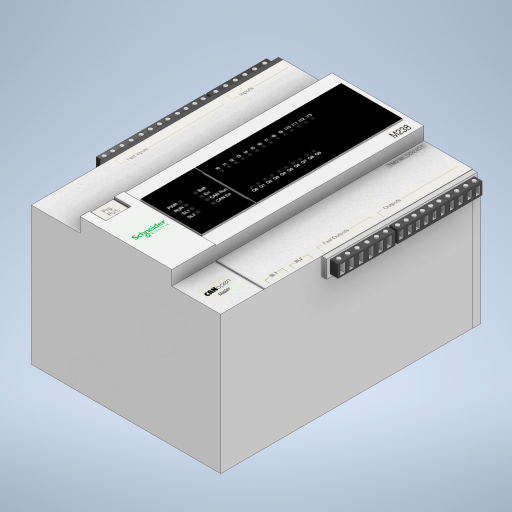
# Autodesk Inventor part: PLC
Saved by Autodesk Inventor 2023 (Build 270158000, 158)
## iProperties
Created: 2022-07-08
Part Number: PLC
Material: Generic
Document SubType Name: Sheet Metal
Designer: User
Density: 1 g/cm^3
Sheet Metal Rule: Default
Appearance: Default
Author: User
Autodesk Inventor part; units mm, degrees
ref_plane "YZ Plane" through (0, 0, 0) normal (1, 0, 0) x (0, 1, 0)
ref_plane "XZ Plane" through (0, 0, 0) normal (0, 1, 0) x (-1, 0, 0)
ref_plane "XY Plane" through (0, 0, 0) normal (0, 0, 1) x (1, 0, 0)
sketch "Sketch1" plane through (0, 0, 0) normal (0, 1, 0) x (-1, 0, 0)
  line L0 (-59, -78.5) -> (59, -78.5)
  line L1 (59, -78.5) -> (59, 78.5)
  line L2 (59, 78.5) -> (-59, 78.5)
  line L3 (-59, 78.5) -> (-59, -78.5)
  line L4 (-59, -78.5) -> (59, 78.5) construction
  line L5 (59, -78.5) -> (-59, 78.5) construction
  point P0 (0, 0)
  constraints: 12 end point, 2 midpoint, 2 parallel, 1 horizontal, 1 perpendicular
extrude "Extrusion1" add sketch "Sketch1" along normal blind 86
sketch "Sketch2" plane through (0, 86, 0) normal (0, 1, 0) x (1, 0, 0)
  line L0 (-59, -78.5) -> (59, -78.5) projected
  line L1 (28.5872, 78.5) -> (-28.5872, 78.5)
  line L2 (-28.5872, 78.5) -> (-28.5872, -78.5)
  line L3 (-28.5872, -78.5) -> (28.5872, -78.5)
  line L4 (28.5872, -78.5) -> (28.5872, 78.5)
  line L5 (28.5872, 78.5) -> (-28.5872, -78.5) construction
  line L6 (-28.5872, 78.5) -> (28.5872, -78.5) construction
  point P0 (0, 0)
  constraints: 12 end point, 2 midpoint, 2 parallel, 1 horizontal, 1 perpendicular, 1 point on line
extrude "Extrusion2" add sketch "Sketch2" along normal blind 8
sketch "Sketch3" plane through (0, 94, 0) normal (0, 1, 0) x (1, 0, 0)
  line L0 (-28.5872, 78.5) -> (-28.5872, -78.5) projected
  line L1 (28.5872, -51.4185) -> (-28.5872, -51.4185)
  line L2 (-28.5872, -51.4185) -> (-28.5872, -78.5)
  line L3 (-28.5872, -78.5) -> (28.5872, -78.5)
  line L4 (28.5872, -78.5) -> (28.5872, -51.4185)
  line L5 (28.5872, -51.4185) -> (-28.5872, -78.5) construction
  line L6 (-28.5872, -51.4185) -> (28.5872, -78.5) construction
  line L7 (-19.1432, -51.4185) -> (19.1432, -51.4185)
  line L8 (18.8938, 74.8007) -> (-19.149, 74.8007)
  line L9 (-19.149, 74.8007) -> (-19.149, -16.0949)
  line L10 (-19.149, -16.0949) -> (18.8938, -16.0949)
  line L11 (18.8938, -16.0949) -> (18.8938, 74.8007)
  line L12 (18.8938, 74.8007) -> (-19.149, -16.0949) construction
  line L13 (-19.149, 74.8007) -> (18.8938, -16.0949) construction
  line L14 (18.8938, -16.7205) -> (-19.149, -16.7205)
  line L15 (-19.149, -16.7205) -> (-19.149, -50.1614)
  line L16 (-19.149, -50.1614) -> (18.8938, -50.1614)
  line L17 (18.8938, -50.1614) -> (18.8938, -16.7205)
  line L18 (18.8938, -16.7205) -> (-19.149, -50.1614) construction
  line L19 (-19.149, -16.7205) -> (18.8938, -50.1614) construction
  point P0 (0, 0)
  point P1 (0, -64.9593)
  point P2 (-0.1276, 29.3529)
  point P3 (-0.1276, -33.4409)
  constraints: 38 end point, 6 midpoint, 6 parallel, 3 horizontal, 3 perpendicular, 1 point on line
extrude "Extrusion3" add sketch "Sketch3" along normal blind 1 contours L11 L10 L9 L8
extrude "Extrusion4" add sketch "Sketch3" along normal blind 1 contours L17 L16 L15 L14
extrude "Extrusion5" add sketch "Sketch3" along normal blind 1 contours L1 L4 L3 L0
sketch "Sketch4" plane through (0, 95, 0) normal (0, 1, 0) x (1, 0, 0)
  line L0 (-28.5872, -78.5) -> (-28.5872, 78.5) projected
  line L1 (-18.1707, -57.2784) -> (-28.5872, -57.2784)
  line L2 (-28.5872, -57.2784) -> (-28.5872, -72.8644)
  line L3 (-28.5872, -72.8644) -> (-18.1707, -72.8644)
  line L4 (-18.1707, -72.8644) -> (-18.1707, -57.2784)
  line L5 (-18.1707, -57.2784) -> (-28.5872, -72.8644) construction
  line L6 (-28.5872, -57.2784) -> (-18.1707, -72.8644) construction
  point P0 (0, 0)
  point P1 (-23.379, -65.0714)
  constraints: 12 end point, 2 midpoint, 2 parallel, 1 horizontal, 1 perpendicular, 1 point on line
extrude "Extrusion6" cut sketch "Sketch4" against normal blind 1
sketch "Sketch5" plane through (-59, 0, -78.5) normal (-1, 0, 0) x (0, 0, 1)
  line L0 (-0.0793, 85.7228) -> (111.1007, 85.7228)
  line L1 (111.1007, 85.7228) -> (111.1007, 74.8127)
  line L2 (111.1007, 74.8127) -> (-0.0793, 74.8127)
  line L3 (-0.0793, 74.8127) -> (-0.0793, 85.7228)
  line L4 (-0.0793, 85.7228) -> (111.1007, 74.8127) construction
  line L5 (111.1007, 85.7228) -> (-0.0793, 74.8127) construction
  point P0 (78.5, 0)
  point P1 (55.5107, 80.2677)
  dimension "d270" = 10.9102
  constraints: 12 end point, 2 midpoint, 2 parallel, 1 horizontal, 1 perpendicular
  measures "d270" distance of L0.end L1.end
extrude "Extrusion7" add sketch "Sketch5" along normal blind 3
sketch "Sketch6" plane through (-62, 0, -78.5) normal (-1, 0, 0) x (0, 0, 1)
  line L0 (40.9569, 76.775) -> (108.5085, 76.775)
  line L1 (108.5085, 76.775) -> (108.5085, 83.79)
  line L2 (108.5085, 83.79) -> (40.9569, 83.79)
  line L3 (40.9569, 83.79) -> (40.9569, 76.775)
  line L4 (40.9569, 76.775) -> (108.5085, 83.79) construction
  line L5 (108.5085, 76.775) -> (40.9569, 83.79) construction
  line L6 (2.4823, 83.7437) -> (39.9398, 83.7437)
  line L7 (39.9398, 83.7437) -> (39.9398, 76.8213)
  line L8 (39.9398, 76.8213) -> (2.4823, 76.8213)
  line L9 (2.4823, 76.8213) -> (2.4823, 83.7437)
  line L10 (2.4823, 83.7437) -> (39.9398, 76.8213) construction
  line L11 (39.9398, 83.7437) -> (2.4823, 76.8213) construction
  point P0 (78.5, 0)
  point P1 (74.7327, 80.2825)
  point P2 (21.211, 80.2825)
  constraints: 24 end point, 4 midpoint, 4 parallel, 2 horizontal, 2 perpendicular
extrude "Extrusion8" add sketch "Sketch6" along normal blind 5 contours L3 L2 L1 L0
extrude "Extrusion9" add sketch "Sketch6" along normal blind 5 contours L6 L7 L8 L9
sketch "Sketch7" plane through (-62, 83.79, 30.0085) normal (0, 1, 0) x (1, 0, 0)
  circle A0 centre (-2.5704, 2.5116) radius 1.27
  circle A1 centre (-2.5676, 7.7493) radius 1.27
  circle A2 centre (-2.5676, 19.2576) radius 1.27
  circle A3 centre (-2.5676, 13.5035) radius 1.27
  circle A4 centre (-2.5676, 25.5282) radius 1.27
  circle A5 centre (-2.5676, 31.3561) radius 1.27
  circle A6 centre (-2.5676, 42.1267) radius 1.27
  circle A7 centre (-2.5676, 36.9627) radius 1.27
  circle A8 centre (-2.5676, 48.1759) radius 1.27
  circle A9 centre (-2.5676, 53.4874) radius 1.27
  circle A10 centre (-2.5676, 64.1678) radius 1.27
  circle A11 centre (-2.5676, 58.9465) radius 1.27
  point P0 (62, 30.0085)
  dimension "d20" = 2.54
  dimension "d21" = 2.54
  dimension "d22" = 2.54
  dimension "d23" = 2.54
  dimension "d24" = 2.54
  dimension "d25" = 2.54
  dimension "d26" = 2.54
  dimension "d27" = 2.54
  dimension "d28" = 2.54
  dimension "d29" = 2.54
  dimension "d30" = 2.54
  dimension "d31" = 2.54
  constraints: 12 centre point
  measures "d20" diameter of A0
  measures "d21" diameter of A1
  measures "d22" diameter of A2
  measures "d23" diameter of A3
  measures "d24" diameter of A4
  measures "d25" diameter of A5
  measures "d26" diameter of A6
  measures "d27" diameter of A7
  measures "d28" diameter of A8
  measures "d29" diameter of A9
  measures "d30" diameter of A10
  measures "d31" diameter of A11
extrude "Extrusion10" add sketch "Sketch7" along normal blind 0.5 contours A0
extrude "Extrusion11" add sketch "Sketch7" along normal blind 0.5 contours A1
extrude "Extrusion12" add sketch "Sketch7" along normal blind 0.5 contours A3
extrude "Extrusion13" add sketch "Sketch7" along normal blind 0.5 contours A2
extrude "Extrusion14" add sketch "Sketch7" along normal blind 0.5 contours A4
extrude "Extrusion15" add sketch "Sketch7" along normal blind 0.5 contours A5
extrude "Extrusion16" add sketch "Sketch7" along normal blind 0.5 contours A7
extrude "Extrusion17" add sketch "Sketch7" along normal blind 0.5 contours A6
extrude "Extrusion18" add sketch "Sketch7" along normal blind 0.5 contours A8
extrude "Extrusion19" add sketch "Sketch7" along normal blind 0.5 contours A9
extrude "Extrusion20" add sketch "Sketch7" along normal blind 0.5 contours A11
extrude "Extrusion21" add sketch "Sketch7" along normal blind 0.5 contours A10
sketch "Sketch8" plane through (-62, 83.7437, -38.5602) normal (0, 1, 0) x (1, 0, 0)
  circle A0 centre (-2.5305, 3.4573) radius 1.27
  circle A1 centre (-2.5952, 9.6724) radius 1.27
  circle A2 centre (-2.5952, 21.6396) radius 1.27
  circle A3 centre (-2.5952, 15.689) radius 1.27
  circle A4 centre (-2.5952, 27.7224) radius 1.27
  circle A5 centre (-2.5952, 34.0035) radius 1.27
  point P0 (62, -38.5602)
  dimension "d56" = 2.54
  dimension "d57" = 2.54
  dimension "d58" = 2.54
  dimension "d59" = 2.54
  dimension "d60" = 2.54
  dimension "d61" = 2.54
  constraints: 6 centre point
  measures "d56" diameter of A0
  measures "d57" diameter of A1
  measures "d58" diameter of A2
  measures "d59" diameter of A3
  measures "d60" diameter of A4
  measures "d61" diameter of A5
extrude "Extrusion22" add sketch "Sketch8" along normal blind 0.5 contours A0
extrude "Extrusion23" add sketch "Sketch8" along normal blind 0.5 contours A1
extrude "Extrusion24" add sketch "Sketch8" along normal blind 0.5 contours A3
extrude "Extrusion25" add sketch "Sketch8" along normal blind 0.5 contours A2
extrude "Extrusion26" add sketch "Sketch8" along normal blind 0.5 contours A4
extrude "Extrusion27" add sketch "Sketch8" along normal blind 0.5 contours A5
sketch "Sketch9" plane through (0, 95, 0) normal (0, 1, 0) x (1, 0, 0)
  line L0 (-10.1047, -53.1992) -> (11.9504, -53.1992) construction
  line L1 (11.9504, -53.1992) -> (11.9504, -75.483) construction
  line L2 (11.9504, -75.483) -> (-10.1047, -75.483) construction
  line L3 (-10.1047, -75.483) -> (-10.1047, -53.1992) construction
  point P0 (0, 0)
  constraints: 2 other
decal "Decal1"
sketch "Sketch10" plane through (0, 95, 0) normal (0, 1, 0) x (1, 0, 0)
  line L0 (-13.6554, -16.7848) -> (14.4275, -16.7848) construction
  line L1 (14.4275, -16.7848) -> (14.4275, -50.0682) construction
  line L2 (14.4275, -50.0682) -> (-13.6554, -50.0682) construction
  line L3 (-13.6554, -50.0682) -> (-13.6554, -16.7848) construction
  line L4 (21.6211, 74.4866) -> (26.8689, 74.4866) construction
  line L5 (26.8689, 74.4866) -> (26.8689, 61.9983) construction
  line L6 (26.8689, 61.9983) -> (21.6211, 61.9983) construction
  line L7 (21.6211, 61.9983) -> (21.6211, 74.4866) construction
  line L8 (-58.2252, 36.6989) -> (-51.617, 36.6989) construction
  line L9 (-51.617, 36.6989) -> (-51.617, -29.4508) construction
  line L10 (-51.617, -29.4508) -> (-58.2252, -29.4508) construction
  line L11 (-58.2252, -29.4508) -> (-58.2252, 36.6989) construction
  point P0 (0, 0)
  constraints: 6 other
decal "Decal2"
decal "Decal3"
decal "Decal4"
sketch "Sketch11" plane through (0, 86, 0) normal (0, 1, 0) x (1, 0, 0)
  line L0 (29.6735, 76.7479) -> (33.1381, 76.7479) construction
  line L1 (33.1381, 76.7479) -> (33.1381, 52.8308) construction
  line L2 (33.1381, 52.8308) -> (29.6735, 52.8308) construction
  line L3 (29.6735, 52.8308) -> (29.6735, 76.7479) construction
  point P0 (0, 0)
  constraints: 2 other
decal "Decal5"
sketch "Sketch12" plane through (0, 86, 0) normal (0, 1, 0) x (1, 0, 0)
  line L0 (-58.554, 77.2781) -> (-50.311, 77.2781) construction
  line L1 (-50.311, 77.2781) -> (-50.311, 39.3956) construction
  line L2 (-50.311, 39.3956) -> (-58.554, 39.3956) construction
  line L3 (-58.554, 39.3956) -> (-58.554, 77.2781) construction
  point P0 (0, 0)
  constraints: 2 other
decal "Decal6"
sketch "Sketch13" plane through (59, 0, 78.5) normal (1, 0, 0) x (0, 0, -1)
  line L0 (156.8045, 74.8146) -> (63.0543, 74.8146)
  line L1 (63.0543, 74.8146) -> (63.0543, 85.7366)
  line L2 (63.0543, 85.7366) -> (156.8045, 85.7366)
  line L3 (156.8045, 85.7366) -> (156.8045, 74.8146)
  line L4 (156.8045, 74.8146) -> (63.0543, 85.7366) construction
  line L5 (63.0543, 74.8146) -> (156.8045, 85.7366) construction
  point P0 (78.5, 0)
  point P1 (109.9294, 80.2756)
  constraints: 12 end point, 2 midpoint, 2 parallel, 1 horizontal, 1 perpendicular
extrude "Extrusion28" add sketch "Sketch13" along normal blind 3
sketch "Sketch14" plane through (62, 86, 0) normal (1, 0, 0) x (0, -1, 0)
  line L0 (9.3005, -13.3278) -> (1.4582, -13.3278)
  line L1 (1.4582, -13.3278) -> (1.4582, 22.2214)
  line L2 (1.4582, 22.2214) -> (9.3005, 22.2214)
  line L3 (9.3005, 22.2214) -> (9.3005, -13.3278)
  line L4 (9.3005, -13.3278) -> (1.4582, 22.2214) construction
  line L5 (1.4582, -13.3278) -> (9.3005, 22.2214) construction
  line L6 (1.5726, 23.7364) -> (9.1861, 23.7364)
  line L7 (9.1861, 23.7364) -> (9.1861, 76.506)
  line L8 (9.1861, 76.506) -> (1.5726, 76.506)
  line L9 (1.5726, 76.506) -> (1.5726, 23.7364)
  line L10 (1.5726, 23.7364) -> (9.1861, 76.506) construction
  line L11 (9.1861, 23.7364) -> (1.5726, 76.506) construction
  point P0 (86, 0)
  point P1 (5.3794, 4.4468)
  point P2 (5.3794, 50.1212)
  constraints: 24 end point, 4 midpoint, 4 parallel, 2 horizontal, 2 perpendicular
extrude "Extrusion29" add sketch "Sketch14" along normal blind 5 contours L0 L1 L2 L3
extrude "Extrusion30" add sketch "Sketch14" along normal blind 5 contours L9 L8 L7 L6
sketch "Sketch15" plane through (62, 84.5418, 13.3278) normal (0, 1, 0) x (1, 0, 0)
  circle A0 centre (2.4904, 2.9128) radius 1.27
  circle A1 centre (2.4904, 8.3521) radius 1.27
  circle A2 centre (2.4904, 14.2858) radius 1.27
  circle A3 centre (2.4904, 20.4668) radius 1.27
  circle A4 centre (2.4904, 26.4006) radius 1.27
  circle A5 centre (2.4904, 32.0253) radius 1.27
  point P0 (-62, 13.3278)
  dimension "d278" = 2.54
  dimension "d279" = 2.54
  dimension "d280" = 2.54
  dimension "d281" = 2.54
  dimension "d282" = 2.54
  dimension "d283" = 2.54
  constraints: 6 centre point
  measures "d278" diameter of A0
  measures "d279" diameter of A1
  measures "d280" diameter of A2
  measures "d281" diameter of A3
  measures "d282" diameter of A4
  measures "d283" diameter of A5
extrude "Extrusion31" add sketch "Sketch15" along normal blind 0.5 contours A0
extrude "Extrusion32" add sketch "Sketch15" along normal blind 0.5 contours A1
extrude "Extrusion33" add sketch "Sketch15" along normal blind 0.5 contours A2
extrude "Extrusion34" add sketch "Sketch15" along normal blind 0.5 contours A3
extrude "Extrusion35" add sketch "Sketch15" along normal blind 0.5 contours A4
extrude "Extrusion36" add sketch "Sketch15" along normal blind 0.5 contours A5
sketch "Sketch16" plane through (62, 84.4274, -23.7364) normal (0, 1, 0) x (1, 0, 0)
  circle A0 centre (2.6563, 2.3164) radius 1.27
  circle A1 centre (2.6563, 7.6321) radius 1.27
  circle A2 centre (2.6563, 12.5769) radius 1.27
  circle A3 centre (2.6563, 17.7689) radius 1.27
  circle A4 centre (2.6563, 22.8991) radius 1.27
  circle A5 centre (2.6563, 28.0912) radius 1.27
  circle A6 centre (2.6563, 33.5922) radius 1.27
  circle A7 centre (2.6563, 39.1551) radius 1.27
  circle A8 centre (2.6563, 44.7798) radius 1.27
  circle A9 centre (2.6563, 50.0337) radius 1.27
  point P0 (-62, -23.7364)
  dimension "d296" = 2.54
  dimension "d297" = 2.54
  dimension "d298" = 2.54
  dimension "d299" = 2.54
  dimension "d300" = 2.54
  dimension "d301" = 2.54
  dimension "d302" = 2.54
  dimension "d303" = 2.54
  dimension "d304" = 2.54
  dimension "d305" = 2.54
  constraints: 10 centre point
  measures "d296" diameter of A0
  measures "d297" diameter of A1
  measures "d298" diameter of A2
  measures "d299" diameter of A3
  measures "d300" diameter of A4
  measures "d301" diameter of A5
  measures "d302" diameter of A6
  measures "d303" diameter of A7
  measures "d304" diameter of A8
  measures "d305" diameter of A9
extrude "Extrusion37" add sketch "Sketch16" along normal blind 0.5 contours A0
extrude "Extrusion38" add sketch "Sketch16" along normal blind 0.5 contours A1
extrude "Extrusion39" add sketch "Sketch16" along normal blind 0.5 contours A2
extrude "Extrusion40" add sketch "Sketch16" along normal blind 0.5 contours A3
extrude "Extrusion41" add sketch "Sketch16" along normal blind 0.5 contours A4
extrude "Extrusion42" add sketch "Sketch16" along normal blind 0.5 contours A5
extrude "Extrusion43" add sketch "Sketch16" along normal blind 0.5 contours A6
extrude "Extrusion44" add sketch "Sketch16" along normal blind 0.5 contours A7
extrude "Extrusion45" add sketch "Sketch16" along normal blind 0.5 contours A8
extrude "Extrusion46" add sketch "Sketch16" along normal blind 0.5 contours A9
sketch "Sketch17" plane through (0, 86, 0) normal (0, 1, 0) x (1, 0, 0)
  line L0 (50.4208, 77.1669) -> (57.9021, 77.1669) construction
  line L1 (57.9021, 77.1669) -> (57.9021, 23.3015) construction
  line L2 (57.9021, 23.3015) -> (50.4208, 23.3015) construction
  line L3 (50.4208, 23.3015) -> (50.4208, 77.1669) construction
  line L4 (50.1649, 22.395) -> (58.1661, 22.395) construction
  line L5 (58.1661, 22.395) -> (58.1661, -14.0662) construction
  line L6 (58.1661, -14.0662) -> (50.1649, -14.0662) construction
  line L7 (50.1649, -14.0662) -> (50.1649, 22.395) construction
  point P0 (0, 0)
  constraints: 4 other
decal "Decal7"
decal "Decal8"
sketch "Sketch18" plane through (0, 95, 0) normal (0, 1, 0) x (1, 0, 0)
  line L0 (-16.2341, 72.1064) -> (15.9464, 72.1064) construction
  line L1 (15.9464, 72.1064) -> (15.9464, -14.584) construction
  line L2 (15.9464, -14.584) -> (-16.2341, -14.584) construction
  line L3 (-16.2341, -14.584) -> (-16.2341, 72.1064) construction
  point P0 (0, 0)
  constraints: 2 other
decal "Decal9"
sketch "Sketch19" plane through (59, 0, -78.5) normal (0, 0, -1) x (-1, 0, 0)
  line L0 (0.0162, 74.5415) -> (117.9838, 74.5415)
  line L1 (117.9838, 74.5415) -> (117.9838, -0.0836)
  line L2 (117.9838, -0.0836) -> (0.0162, -0.0836)
  line L3 (0.0162, -0.0836) -> (0.0162, 74.5415)
  line L4 (0.0162, 74.5415) -> (117.9838, -0.0836) construction
  line L5 (117.9838, 74.5415) -> (0.0162, -0.0836) construction
  point P0 (59, 0)
  point P1 (59, 37.229)
  constraints: 12 end point, 2 midpoint, 2 parallel, 1 horizontal, 1 perpendicular
extrude "Extrusion47" add sketch "Sketch19" along normal blind 5
sketch "Sketch20" plane through (-67, 0, -78.5) normal (-1, 0, 0) x (0, 0, 1)
  line L0 (107.1255, 82.555) -> (104.7702, 82.555)
  line L1 (104.7702, 82.555) -> (104.7702, 78.0406)
  line L2 (104.7702, 78.0406) -> (107.1255, 78.0406)
  line L3 (107.1255, 78.0406) -> (107.1255, 82.555)
  line L4 (107.1255, 82.555) -> (104.7702, 78.0406) construction
  line L5 (104.7702, 82.555) -> (107.1255, 78.0406) construction
  line L6 (102.2296, 78.0852) -> (99.7509, 78.0852)
  line L7 (99.7509, 78.0852) -> (99.7509, 82.5104)
  line L8 (99.7509, 82.5104) -> (102.2296, 82.5104)
  line L9 (102.2296, 82.5104) -> (102.2296, 78.0852)
  line L10 (102.2296, 78.0852) -> (99.7509, 82.5104) construction
  line L11 (99.7509, 78.0852) -> (102.2296, 82.5104) construction
  line L12 (96.3367, 78.063) -> (93.6848, 78.063)
  line L13 (93.6848, 78.063) -> (93.6848, 82.5326)
  line L14 (93.6848, 82.5326) -> (96.3367, 82.5326)
  line L15 (96.3367, 82.5326) -> (96.3367, 78.063)
  line L16 (96.3367, 78.063) -> (93.6848, 82.5326) construction
  line L17 (93.6848, 78.063) -> (96.3367, 82.5326) construction
  line L18 (90.8512, 78.0898) -> (88.1425, 78.0898)
  line L19 (88.1425, 78.0898) -> (88.1425, 82.5058)
  line L20 (88.1425, 82.5058) -> (90.8512, 82.5058)
  line L21 (90.8512, 82.5058) -> (90.8512, 78.0898)
  line L22 (90.8512, 78.0898) -> (88.1425, 82.5058) construction
  line L23 (88.1425, 78.0898) -> (90.8512, 82.5058) construction
  line L24 (84.4554, 78.0406) -> (81.7075, 78.0406)
  line L25 (81.7075, 78.0406) -> (81.7075, 82.555)
  line L26 (81.7075, 82.555) -> (84.4554, 82.555)
  line L27 (84.4554, 82.555) -> (84.4554, 78.0406)
  line L28 (84.4554, 78.0406) -> (81.7075, 82.555) construction
  line L29 (81.7075, 78.0406) -> (84.4554, 82.555) construction
  line L30 (78.5647, 82.744) -> (75.8543, 82.744)
  line L31 (75.8543, 82.744) -> (75.8543, 78.3053)
  line L32 (75.8543, 78.3053) -> (78.5647, 78.3053)
  line L33 (78.5647, 78.3053) -> (78.5647, 82.744)
  line L34 (78.5647, 82.744) -> (75.8543, 78.3053) construction
  line L35 (75.8543, 82.744) -> (78.5647, 78.3053) construction
  line L36 (73.1672, 78.1595) -> (70.2252, 78.1595)
  line L37 (70.2252, 78.1595) -> (70.2252, 82.744)
  line L38 (70.2252, 82.744) -> (73.1672, 82.744)
  line L39 (73.1672, 82.744) -> (73.1672, 78.1595)
  line L40 (73.1672, 78.1595) -> (70.2252, 82.744) construction
  line L41 (70.2252, 78.1595) -> (73.1672, 82.744) construction
  line L42 (65.4366, 82.5982) -> (67.8698, 82.5982)
  line L43 (67.8698, 82.5982) -> (67.8698, 78.3053)
  line L44 (67.8698, 78.3053) -> (65.4366, 78.3053)
  line L45 (65.4366, 78.3053) -> (65.4366, 82.5982)
  line L46 (65.4366, 82.5982) -> (67.8698, 78.3053) construction
  line L47 (67.8698, 82.5982) -> (65.4366, 78.3053) construction
  line L48 (59.1355, 82.5982) -> (61.6871, 82.5982)
  line L49 (61.6871, 82.5982) -> (61.6871, 78.3053)
  line L50 (61.6871, 78.3053) -> (59.1355, 78.3053)
  line L51 (59.1355, 78.3053) -> (59.1355, 82.5982)
  line L52 (59.1355, 82.5982) -> (61.6871, 78.3053) construction
  line L53 (61.6871, 82.5982) -> (59.1355, 78.3053) construction
  line L54 (48.5435, 82.8095) -> (51.0951, 82.8095)
  line L55 (51.0951, 82.8095) -> (51.0951, 78.4731)
  line L56 (51.0951, 78.4731) -> (48.5435, 78.4731)
  line L57 (48.5435, 78.4731) -> (48.5435, 82.8095)
  line L58 (48.5435, 82.8095) -> (51.0951, 78.4731) construction
  line L59 (51.0951, 82.8095) -> (48.5435, 78.4731) construction
  line L60 (43.0921, 82.7647) -> (45.5408, 82.7647)
  line L61 (45.5408, 82.7647) -> (45.5408, 78.5179)
  line L62 (45.5408, 78.5179) -> (43.0921, 78.5179)
  line L63 (43.0921, 78.5179) -> (43.0921, 82.7647)
  line L64 (43.0921, 82.7647) -> (45.5408, 78.5179) construction
  line L65 (45.5408, 82.7647) -> (43.0921, 78.5179) construction
  line L66 (56.2786, 76.6995) -> (56.2786, 84.5418) projected
  line L67 (53.2485, 82.7234) -> (56.2786, 82.7234)
  line L68 (56.2786, 82.7234) -> (56.2786, 78.5179)
  line L69 (56.2786, 78.5179) -> (53.2485, 78.5179)
  line L70 (53.2485, 78.5179) -> (53.2485, 82.7234)
  line L71 (54.7636, 84.4274) -> (54.7636, 76.8139) projected
  line L72 (53.2485, 82.7234) -> (56.2786, 78.5179) construction
  line L73 (56.2786, 82.7234) -> (53.2485, 78.5179) construction
  point P0 (78.5, 0)
  point P1 (105.9478, 80.2978)
  point P2 (100.9903, 80.2978)
  point P3 (95.0108, 80.2978)
  point P4 (89.4968, 80.2978)
  point P5 (83.0814, 80.2978)
  point P6 (77.2095, 80.5246)
  point P7 (71.6962, 80.4517)
  point P8 (66.6532, 80.4517)
  point P9 (60.4113, 80.4517)
  point P10 (49.8193, 80.6413)
  point P11 (44.3165, 80.6413)
  point P12 (54.7636, 80.6206)
  point P13 (54.7636, 78.5179)
  point P14 (54.7636, 82.7234)
  constraints: 144 end point, 25 midpoint, 24 parallel, 12 horizontal, 12 perpendicular, 2 point on line
extrude "Extrusion48" cut sketch "Sketch20" against normal blind 4 contours L3 L2 L1 L0
extrude "Extrusion49" cut sketch "Sketch20" against normal blind 4 contours L6 L7 L8 L9
extrude "Extrusion50" cut sketch "Sketch20" against normal blind 4 contours L12 L13 L14 L15
extrude "Extrusion51" cut sketch "Sketch20" against normal blind 4 contours L18 L19 L20 L21
extrude "Extrusion52" cut sketch "Sketch20" against normal blind 4 contours L24 L25 L26 L27
extrude "Extrusion53" cut sketch "Sketch20" against normal blind 4 contours L33 L32 L31 L30
extrude "Extrusion54" cut sketch "Sketch20" against normal blind 4 contours L36 L37 L38 L39
extrude "Extrusion55" cut sketch "Sketch20" against normal blind 4 contours L42 L43 L44 L45
extrude "Extrusion56" cut sketch "Sketch20" against normal blind 4 contours L48 L49 L50 L51
extrude "Extrusion57" cut sketch "Sketch20" against normal blind 4 contours L69 L70 L67 L71
extrude "Extrusion58" cut sketch "Sketch20" against normal blind 4 contours L69 L71 L67 L66
extrude "Extrusion59" cut sketch "Sketch20" against normal blind 4 contours L54 L55 L56 L57
extrude "Extrusion60" cut sketch "Sketch20" against normal blind 4 contours L60 L61 L62 L63
sketch "Sketch21" plane through (-67, 0, -78.5) normal (-1, 0, 0) x (0, 0, 1)
  line L0 (35.0939, 83.0672) -> (37.8762, 83.0672)
  line L1 (37.8762, 83.0672) -> (37.8762, 77.7742)
  line L2 (37.8762, 77.7742) -> (35.0939, 77.7742)
  line L3 (35.0939, 77.7742) -> (35.0939, 83.0672)
  line L4 (35.0939, 83.0672) -> (37.8762, 77.7742) construction
  line L5 (37.8762, 83.0672) -> (35.0939, 77.7742) construction
  line L6 (31.7697, 77.7742) -> (28.9875, 77.7742)
  line L7 (28.9875, 77.7742) -> (28.9875, 83.0672)
  line L8 (28.9875, 83.0672) -> (31.7697, 83.0672)
  line L9 (31.7697, 83.0672) -> (31.7697, 77.7742)
  line L10 (31.7697, 77.7742) -> (28.9875, 83.0672) construction
  line L11 (28.9875, 77.7742) -> (31.7697, 83.0672) construction
  line L12 (25.5597, 77.7742) -> (23.0489, 77.7742)
  line L13 (23.0489, 77.7742) -> (23.0489, 83.0672)
  line L14 (23.0489, 83.0672) -> (25.5597, 83.0672)
  line L15 (25.5597, 83.0672) -> (25.5597, 77.7742)
  line L16 (25.5597, 77.7742) -> (23.0489, 83.0672) construction
  line L17 (23.0489, 77.7742) -> (25.5597, 83.0672) construction
  line L18 (19.622, 77.7742) -> (16.9755, 77.7742)
  line L19 (16.9755, 77.7742) -> (16.9755, 83.0672)
  line L20 (16.9755, 83.0672) -> (19.622, 83.0672)
  line L21 (19.622, 83.0672) -> (19.622, 77.7742)
  line L22 (19.622, 77.7742) -> (16.9755, 83.0672) construction
  line L23 (16.9755, 77.7742) -> (19.622, 83.0672) construction
  line L24 (13.6504, 77.7742) -> (11.0039, 77.7742)
  line L25 (11.0039, 77.7742) -> (11.0039, 83.0672)
  line L26 (11.0039, 83.0672) -> (13.6504, 83.0672)
  line L27 (13.6504, 83.0672) -> (13.6504, 77.7742)
  line L28 (13.6504, 77.7742) -> (11.0039, 83.0672) construction
  line L29 (11.0039, 77.7742) -> (13.6504, 83.0672) construction
  line L30 (7.3395, 77.7742) -> (4.6251, 77.7742)
  line L31 (4.6251, 77.7742) -> (4.6251, 83.0672)
  line L32 (4.6251, 83.0672) -> (7.3395, 83.0672)
  line L33 (7.3395, 83.0672) -> (7.3395, 77.7742)
  line L34 (7.3395, 77.7742) -> (4.6251, 83.0672) construction
  line L35 (4.6251, 77.7742) -> (7.3395, 83.0672) construction
  point P0 (78.5, 0)
  point P1 (36.485, 80.4207)
  point P2 (30.3786, 80.4207)
  point P3 (24.3043, 80.4207)
  point P4 (18.2988, 80.4207)
  point P5 (12.3272, 80.4207)
  point P6 (5.9823, 80.4207)
  constraints: 72 end point, 12 midpoint, 12 parallel, 6 horizontal, 6 perpendicular, 3 point on line
extrude "Extrusion61" cut sketch "Sketch21" against normal blind 4 contours L0 L1 L2 L3
extrude "Extrusion62" cut sketch "Sketch21" against normal blind 4 contours L6 L7 L8 L9
extrude "Extrusion63" cut sketch "Sketch21" against normal blind 4 contours L12 L13 L14 L15
extrude "Extrusion64" cut sketch "Sketch21" against normal blind 4 contours L18 L19 L20 L21
extrude "Extrusion65" cut sketch "Sketch21" against normal blind 4 contours L24 L25 L26 L27
extrude "Extrusion66" cut sketch "Sketch21" against normal blind 4 contours L30 L31 L32 L33
sketch "Sketch22" plane through (67, 86, 0) normal (1, 0, 0) x (0, 0, -1)
  line L0 (-11.9749, -2.376) -> (-8.9475, -2.376)
  line L1 (-8.9475, -2.376) -> (-8.9475, -8.4309)
  line L2 (-8.9475, -8.4309) -> (-11.9749, -8.4309)
  line L3 (-11.9749, -8.4309) -> (-11.9749, -2.376)
  line L4 (-11.9749, -2.376) -> (-8.9475, -8.4309) construction
  line L5 (-8.9475, -2.376) -> (-11.9749, -8.4309) construction
  line L6 (-6.5226, -2.376) -> (-3.5286, -2.376)
  line L7 (-3.5286, -2.376) -> (-3.5286, -8.4309)
  line L8 (-3.5286, -8.4309) -> (-6.5226, -8.4309)
  line L9 (-6.5226, -8.4309) -> (-6.5226, -2.376)
  line L10 (-6.5226, -2.376) -> (-3.5286, -8.4309) construction
  line L11 (-3.5286, -2.376) -> (-6.5226, -8.4309) construction
  line L12 (-0.3577, -2.3822) -> (2.5081, -2.3822)
  line L13 (2.5081, -2.3822) -> (2.5081, -8.4309)
  line L14 (2.5081, -8.4309) -> (-0.3577, -8.4309)
  line L15 (-0.3577, -8.4309) -> (-0.3577, -2.3822)
  line L16 (-0.3577, -2.3822) -> (2.5081, -8.4309) construction
  line L17 (2.5081, -2.3822) -> (-0.3577, -8.4309) construction
  line L18 (8.6668, -8.4309) -> (5.9145, -8.4309)
  line L19 (5.9145, -8.4309) -> (5.9145, -2.3822)
  line L20 (5.9145, -2.3822) -> (8.6668, -2.3822)
  line L21 (8.6668, -2.3822) -> (8.6668, -8.4309)
  line L22 (8.6668, -8.4309) -> (5.9145, -2.3822) construction
  line L23 (5.9145, -8.4309) -> (8.6668, -2.3822) construction
  line L24 (14.6609, -8.4309) -> (11.8468, -8.4309)
  line L25 (11.8468, -8.4309) -> (11.8468, -2.3822)
  line L26 (11.8468, -2.3822) -> (14.6609, -2.3822)
  line L27 (14.6609, -2.3822) -> (14.6609, -8.4309)
  line L28 (14.6609, -8.4309) -> (11.8468, -2.3822) construction
  line L29 (11.8468, -8.4309) -> (14.6609, -2.3822) construction
  line L30 (20.1344, -8.4309) -> (17.3363, -8.4309)
  line L31 (17.3363, -8.4309) -> (17.3363, -2.3822)
  line L32 (17.3363, -2.3822) -> (20.1344, -2.3822)
  line L33 (20.1344, -2.3822) -> (20.1344, -8.4309)
  line L34 (20.1344, -8.4309) -> (17.3363, -2.3822) construction
  line L35 (17.3363, -8.4309) -> (20.1344, -2.3822) construction
  point P0 (0, -86)
  point P1 (-10.4612, -5.4035)
  point P2 (-5.0256, -5.4035)
  point P3 (1.0752, -5.4066)
  point P4 (7.2907, -5.4066)
  point P5 (13.2538, -5.4066)
  point P6 (18.7354, -5.4066)
  constraints: 72 end point, 12 midpoint, 12 parallel, 6 horizontal, 6 perpendicular, 4 point on line
extrude "Extrusion67" cut sketch "Sketch22" against normal blind 4 contours L0 L1 L2 L3
extrude "Extrusion68" cut sketch "Sketch22" against normal blind 4 contours L6 L7 L8 L9
extrude "Extrusion69" cut sketch "Sketch22" against normal blind 4 contours L12 L13 L14 L15
extrude "Extrusion70" cut sketch "Sketch22" against normal blind 4 contours L18 L19 L20 L21
extrude "Extrusion71" cut sketch "Sketch22" against normal blind 4 contours L24 L25 L26 L27
extrude "Extrusion72" cut sketch "Sketch22" against normal blind 4 contours L30 L31 L32 L33
sketch "Sketch23" plane through (67, 86, 0) normal (1, 0, 0) x (0, 0, -1)
  line L0 (27.4973, -7.6744) -> (24.7964, -7.6744)
  line L1 (24.7964, -7.6744) -> (24.7964, -2.8473)
  line L2 (24.7964, -2.8473) -> (27.4973, -2.8473)
  line L3 (27.4973, -2.8473) -> (27.4973, -7.6744)
  line L4 (27.4973, -7.6744) -> (24.7964, -2.8473) construction
  line L5 (24.7964, -7.6744) -> (27.4973, -2.8473) construction
  line L6 (32.6979, -7.6744) -> (30.1694, -7.6744)
  line L7 (30.1694, -7.6744) -> (30.1694, -2.8473)
  line L8 (30.1694, -2.8473) -> (32.6979, -2.8473)
  line L9 (32.6979, -2.8473) -> (32.6979, -7.6744)
  line L10 (32.6979, -7.6744) -> (30.1694, -2.8473) construction
  line L11 (30.1694, -7.6744) -> (32.6979, -2.8473) construction
  line L12 (37.7261, -7.6744) -> (35.0827, -7.6744)
  line L13 (35.0827, -7.6744) -> (35.0827, -2.8473)
  line L14 (35.0827, -2.8473) -> (37.7261, -2.8473)
  line L15 (37.7261, -2.8473) -> (37.7261, -7.6744)
  line L16 (37.7261, -7.6744) -> (35.0827, -2.8473) construction
  line L17 (35.0827, -7.6744) -> (37.7261, -2.8473) construction
  line L18 (42.9931, -7.589) -> (40.3499, -7.589)
  line L19 (40.3499, -7.589) -> (40.3499, -3.0321)
  line L20 (40.3499, -3.0321) -> (42.9931, -3.0321)
  line L21 (42.9931, -3.0321) -> (42.9931, -7.589)
  line L22 (42.9931, -7.589) -> (40.3499, -3.0321) construction
  line L23 (40.3499, -7.589) -> (42.9931, -3.0321) construction
  line L24 (47.9857, -7.4897) -> (45.4749, -7.4897)
  line L25 (45.4749, -7.4897) -> (45.4749, -3.0321)
  line L26 (45.4749, -3.0321) -> (47.9857, -3.0321)
  line L27 (47.9857, -3.0321) -> (47.9857, -7.4897)
  line L28 (46.7303, -2.9328) -> (46.7303, -8.2258) projected
  line L29 (47.9857, -7.4897) -> (45.4749, -3.0321) construction
  line L30 (45.4749, -7.4897) -> (47.9857, -3.0321) construction
  line L31 (53.1981, -7.6195) -> (50.6873, -7.6195)
  line L32 (50.6873, -7.6195) -> (50.6873, -2.8171)
  line L33 (50.6873, -2.8171) -> (53.1981, -2.8171)
  line L34 (53.1981, -2.8171) -> (53.1981, -7.6195)
  line L35 (53.1981, -7.6195) -> (50.6873, -2.8171) construction
  line L36 (50.6873, -7.6195) -> (53.1981, -2.8171) construction
  line L37 (58.8147, -7.6519) -> (56.2814, -7.6519)
  line L38 (56.2814, -7.6519) -> (56.2814, -2.8171)
  line L39 (56.2814, -2.8171) -> (58.8147, -2.8171)
  line L40 (58.8147, -2.8171) -> (58.8147, -7.6519)
  line L41 (58.8147, -7.6519) -> (56.2814, -2.8171) construction
  line L42 (56.2814, -7.6519) -> (58.8147, -2.8171) construction
  line L43 (64.4282, -7.5899) -> (61.711, -7.5899)
  line L44 (61.711, -7.5899) -> (61.711, -2.9328)
  line L45 (61.711, -2.9328) -> (64.4282, -2.9328)
  line L46 (64.4282, -2.9328) -> (64.4282, -7.5899)
  line L47 (64.4282, -7.5899) -> (61.711, -2.9328) construction
  line L48 (61.711, -7.5899) -> (64.4282, -2.9328) construction
  line L49 (67.4961, -2.9328) -> (64.8496, -2.9328) projected
  line L50 (70.0196, -7.5362) -> (67.3897, -7.5362)
  line L51 (67.3897, -7.5362) -> (67.3897, -2.9328)
  line L52 (67.3897, -2.9328) -> (70.0196, -2.9328)
  line L53 (70.0196, -2.9328) -> (70.0196, -7.5362)
  line L54 (70.0196, -7.5362) -> (67.3897, -2.9328) construction
  line L55 (67.3897, -7.5362) -> (70.0196, -2.9328) construction
  line L56 (75.178, -7.9836) -> (72.5717, -7.9836)
  line L57 (72.5717, -7.9836) -> (72.5717, -3.175)
  line L58 (72.5717, -3.175) -> (75.178, -3.175)
  line L59 (75.178, -3.175) -> (75.178, -7.9836)
  line L60 (73.8749, -8.2258) -> (73.8749, -2.9328) projected
  line L61 (75.178, -7.9836) -> (72.5717, -3.175) construction
  line L62 (72.5717, -7.9836) -> (75.178, -3.175) construction
  point P0 (0, -86)
  point P1 (26.1468, -5.2609)
  point P2 (31.4337, -5.2609)
  point P3 (36.4044, -5.2609)
  point P4 (41.6715, -5.3105)
  point P5 (46.7303, -5.2609)
  point P6 (51.9427, -5.2183)
  point P7 (57.5481, -5.2345)
  point P8 (63.0696, -5.2614)
  point P9 (68.7046, -5.2345)
  point P10 (73.8749, -5.5793)
  point P11 (46.7303, -3.0321)
  point P12 (46.7303, -7.4897)
  constraints: 118 end point, 21 midpoint, 19 parallel, 11 horizontal, 10 perpendicular, 5 point on line, 3 other
extrude "Extrusion73" cut sketch "Sketch23" against normal blind 4 contours L0 L1 L2 L3
extrude "Extrusion74" cut sketch "Sketch23" against normal blind 4 contours L6 L7 L8 L9
extrude "Extrusion75" cut sketch "Sketch23" against normal blind 4 contours L12 L13 L14 L15
extrude "Extrusion76" cut sketch "Sketch23" against normal blind 4 contours L18 L19 L20 L21
extrude "Extrusion77" cut sketch "Sketch23" against normal blind 4 contours L24 L28 L26 L27
extrude "Extrusion78" cut sketch "Sketch23" against normal blind 4 contours L24 L25 L26 L28
extrude "Extrusion79" cut sketch "Sketch23" against normal blind 4 contours L31 L32 L33 L34
extrude "Extrusion80" cut sketch "Sketch23" against normal blind 4 contours L37 L38 L39 L40
extrude "Extrusion81" cut sketch "Sketch23" against normal blind 4 contours L43 L44 L45 L46
extrude "Extrusion82" cut sketch "Sketch23" against normal blind 4 contours L52 L53 L50 L51 L49
extrude "Extrusion83" cut sketch "Sketch23" against normal blind 4 contours L56 L60 L58 L59 | L56 L57 L58 L60
sketch "Sketch24" plane through (0, 94, 0) normal (0, 1, 0) x (1, 0, 0)
  line L0 (-28.5678, -58.1225) -> (-18.7458, -58.1225) construction
  line L1 (-18.7458, -58.1225) -> (-18.7458, -71.6521) construction
  line L2 (-18.7458, -71.6521) -> (-28.5678, -71.6521) construction
  line L3 (-28.5678, -71.6521) -> (-28.5678, -58.1225) construction
  point P0 (0, 0)
  constraints: 2 other
decal "Decal10"
sketch "Sketch25" plane through (0, 95, 0) normal (0, 1, 0) x (1, 0, 0)
  point P0 (0, 0)
sketch "Sketch26" plane through (0, 86, 0) normal (0, 1, 0) x (1, 0, 0)
  line L0 (39.2807, -55.8995) -> (50.4953, -55.8995) construction
  line L1 (50.4953, -55.8995) -> (50.4953, -74.7003) construction
  line L2 (50.4953, -74.7003) -> (39.2807, -74.7003) construction
  line L3 (39.2807, -74.7003) -> (39.2807, -55.8995) construction
  point P0 (0, 0)
  constraints: 2 other
decal "Decal11"
sketch "Sketch27" plane through (0, 86, 0) normal (0, 1, 0) x (1, 0, 0)
  line L0 (51.6418, -17.4428) -> (57.6891, -17.6709) construction
  line L1 (57.6891, -17.6709) -> (57.1398, -32.2406) construction
  line L2 (57.1398, -32.2406) -> (51.0924, -32.0126) construction
  line L3 (51.0924, -32.0126) -> (51.6418, -17.4428) construction
  line L4 (51.6418, -33.1002) -> (57.4394, -33.1002) construction
  line L5 (57.4394, -33.1002) -> (57.4394, -47.7984) construction
  line L6 (57.4394, -47.7984) -> (51.6418, -47.7984) construction
  line L7 (51.6418, -47.7984) -> (51.6418, -33.1002) construction
  point P0 (0, 0)
  constraints: 4 other
decal "Decal12"
decal "Decal13"
sketch "Sketch28" plane through (0, 86, 0) normal (0, 1, 0) x (1, 0, 0)
  line L0 (58.8355, -50.9932) -> (28.8764, -50.9932)
  line L1 (28.8764, -50.9932) -> (28.8764, -51.7175)
  line L2 (28.8764, -51.7175) -> (58.8355, -51.7175)
  line L3 (58.8355, -51.7175) -> (58.8355, -50.9932)
  line L4 (58.8355, -50.9932) -> (28.8764, -51.7175) construction
  line L5 (28.8764, -50.9932) -> (58.8355, -51.7175) construction
  point P0 (0, 0)
  point P1 (43.856, -51.3554)
  constraints: 12 end point, 2 midpoint, 2 parallel, 1 horizontal, 1 perpendicular
extrude "Extrusion84" cut sketch "Sketch28" against normal blind 2
sketch "Sketch29" plane through (-59, 0, -78.5) normal (-1, 0, 0) x (0, 0, 1)
  line L0 (154.0434, 28.5875) -> (145.7647, 28.5875)
  line L1 (145.7647, 28.5875) -> (145.7647, 5.3036)
  line L2 (145.7647, 5.3036) -> (154.0434, 5.3036)
  line L3 (154.0434, 5.3036) -> (154.0434, 28.5875)
  line L4 (154.0434, 28.5875) -> (145.7647, 5.3036) construction
  line L5 (145.7647, 28.5875) -> (154.0434, 5.3036) construction
  point P0 (78.5, 0)
  point P1 (149.9041, 16.9455)
  constraints: 12 end point, 2 midpoint, 2 parallel, 1 horizontal, 1 perpendicular
extrude "Extrusion85" cut sketch "Sketch29" against normal blind 10
equation "\"BendRadius\" = Thickness"
equation "\"BendReliefWidth\" = Thickness"
equation "\"BendReliefDepth\" = 0.5 * Thickness"
equation "\"CornerReliefSize\" = 4 * Thickness"
equation "\"MinimumRemnant\" = 2 * Thickness"
equation "\"TransitionRadius\" = BendRadius"
equation "\"JacobiRadiusSize\" = BendRadius"
equation "\"GapSize\" = Thickness"
equation "\"Thickness\" = 3.048"
body "Solid1"
